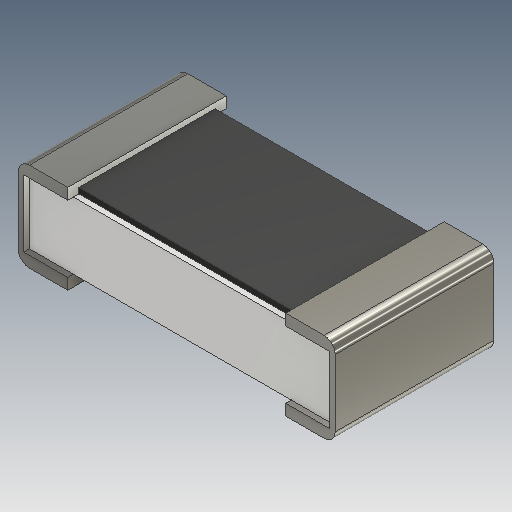
# Autodesk Inventor part: RC0603
Saved by Autodesk Inventor 2018 (Build 220112000, 112)
## iProperties
Created: 2015-10-12
Part Number: RC0603
Material: ABS Plastic
Document SubType Name: Modeling
Designer: Sawaiz
Density: 1.06 g/cm^3
Appearance: Smooth - White
Author: Sawaiz
Autodesk Inventor part; units mm, degrees
ref_plane "YZ Plane" through (0, 0, 0) normal (1, 0, 0) x (0, 1, 0)
ref_plane "XZ Plane" through (0, 0, 0) normal (0, 1, 0) x (-1, 0, 0)
ref_plane "XY Plane" through (0, 0, 0) normal (0, 0, 1) x (1, 0, 0)
sketch "Sketch1" plane through (0, 0, 0) normal (0, 0, 1) x (1, 0, 0)
  line L0 (0.4, -0.8) -> (-0.4, -0.8)
  line L1 (-0.4, -0.8) -> (-0.4, 0.8)
  line L2 (-0.4, 0.8) -> (0.4, 0.8)
  line L3 (0.4, 0.8) -> (0.4, -0.8)
  line L4 (0.4, -0.8) -> (-0.4, 0.8) construction
  line L5 (-0.4, -0.8) -> (0.4, 0.8) construction
  point P0 (0, 0)
  dimension "d0" = 0.8
  dimension "d1" = 1.6
  constraints: 12 end point, 2 midpoint, 2 parallel, 1 horizontal, 1 perpendicular
  measures "d0" distance of L1.end L2.end
  measures "d1" distance of L0.end L1.end
extrude "Extrusion1" add sketch "Sketch1" along normal blind 0.45
sketch "Sketch2" plane through (0, 0, 0) normal (0, 0, -1) x (-1, 0, 0)
  line L0 (-0.4, -0.8) -> (0.4, -0.8) projected
  line L1 (0.4, -0.8) -> (0.4, 0.8) projected
  line L2 (0.4, 0.8) -> (-0.4, 0.8) projected
  line L3 (-0.4, 0.8) -> (-0.4, -0.8) projected
  line L4 (-0.4, -0.55) -> (0.4, -0.55)
  line L5 (0.4, 0.8) -> (0.4, -0.8) projected
  line L6 (0.4, 0.55) -> (-0.4, 0.55)
  point P0 (0, 0)
  dimension "d4" = 0.25
  dimension "d5" = 0.25
  constraints: 4 end point, 4 point on line, 1 horizontal, 1 parallel
  measures "d4" distance between parallel lines of L2 L6
  measures "d5" distance between parallel lines of L0 L4
extrude "Extrusion2" cut sketch "Sketch2" against normal blind 0.0563 contours L3 L6 L1 L4
sketch "Sketch3" plane through (0, 0, 0.45) normal (0, 0, 1) x (1, 0, 0)
  line L0 (-0.4, -0.8) -> (0.4, -0.8) projected
  line L1 (0.4, -0.8) -> (0.4, 0.8) projected
  line L2 (0.4, 0.8) -> (-0.4, 0.8) projected
  line L3 (-0.4, 0.8) -> (-0.4, -0.8) projected
  line L4 (-0.4, 0.55) -> (-0.4, -0.55) projected
  line L5 (-0.4, -0.8) -> (-0.4, 0.8) projected
  line L6 (0.4, 0.8) -> (-0.4, 0.8) projected
  line L7 (0.4, 0.55) -> (-0.4, 0.55)
  line L8 (-0.4, 0.55) -> (-0.4, -0.55)
  line L9 (-0.4, -0.55) -> (0.4, -0.55)
  line L10 (0.4, -0.55) -> (0.4, 0.55)
  line L11 (0.4, 0.55) -> (-0.4, -0.55) construction
  line L12 (-0.4, 0.55) -> (0.4, -0.55) construction
  point P0 (0, 0)
  dimension "d22" = 0.25
  constraints: 12 end point, 2 midpoint, 2 parallel, 1 horizontal, 1 perpendicular, 1 point on line
  measures "d22" distance between parallel lines of L0 L9
extrude "Extrusion7" cut sketch "Sketch3" against normal blind 0.0563 contours L3 L7 L1 L9
sketch "Sketch4" plane through (0.4, -0.8, 0.45) normal (1, 0, 0) x (0, 0, -1)
  line L0 (0, 0) -> (0, 0.25) projected
  line L1 (0.45, 0) -> (0, 0) projected
  line L2 (0.45, 0.25) -> (0.45, 0) projected
  line L3 (0.45, 1.6) -> (0, 1.6) projected
  line L4 (0.45, 0.25) -> (0.3938, 0.25) projected
  line L5 (0.3938, 0.25) -> (0.3938, 1.35) projected
  line L6 (0.3938, 1.35) -> (0.45, 1.35) projected
  line L7 (0.45, 1.6) -> (0.45, 1.35) projected
  line L8 (0.0562, 0.25) -> (0, 0.25) projected
  line L9 (0, 1.35) -> (0.0562, 1.35) projected
  line L10 (0.0562, 1.35) -> (0.0562, 0.25) projected
  line L11 (0.3938, 0.0281) -> (0.0562, 0.0281)
  line L12 (0.0562, 0.0281) -> (0.0562, 1.5719)
  line L13 (0.0562, 1.5719) -> (0.3937, 1.5719)
  line L14 (0.3937, 1.5719) -> (0.3938, 0.0281)
  line L15 (0.3938, 0.0281) -> (0.0562, 1.5719) construction
  line L16 (0.0562, 0.0281) -> (0.3937, 1.5719) construction
  line L17 (0, 1.35) -> (0, 1.6) projected
  point P0 (0.225, 0.8)
  dimension "d25" = 0.0281
  dimension "d26" = 0.0281
  constraints: 12 end point, 2 collinear, 2 midpoint, 2 parallel, 1 horizontal, 1 perpendicular
  measures "d25" distance between parallel lines of L3 L13
  measures "d26" distance between parallel lines of L1 L11
extrude "Extrusion8" cut sketch "Sketch4" against normal blind 0.0281 contours L10 L12 L13 L14 L5 L11
mirror "Mirror1" about plane through (0, 0, 0) normal (1, 0, 0) of "Extrusion8"
sketch "Sketch7" plane through (0, 0, 0.3938) normal (0, 0, 1) x (1, 0, 0)
  line L0 (-0.3719, 0.55) -> (-0.3719, -0.55) projected
  line L1 (0.3719, -0.55) -> (-0.3719, -0.55) projected
  line L2 (0.3719, -0.55) -> (0.3719, 0.55) projected
  line L3 (-0.3719, 0.55) -> (0.3719, 0.55) projected
  point P0 (0, 0)
extrude "Extrusion9" add sketch "Sketch7" along normal blind 0.0281
sketch "Sketch8" plane through (0.3719, -0.8, 0.45) normal (1, 0, 0) x (0, 0, -1)
  line L0 (0.3938, 0.0281) -> (0.0562, 0.0281) projected
  line L1 (0.3938, 0.25) -> (0.3938, 0.0281) projected
  line L2 (0.3937, 1.35) -> (0.3938, 0.25) projected
  line L3 (0.3937, 1.5719) -> (0.3937, 1.35) projected
  line L4 (0.0562, 1.5719) -> (0.3937, 1.5719) projected
  line L5 (0.0562, 1.35) -> (0.0562, 1.5719) projected
  line L6 (0.0281, 1.35) -> (0.0562, 1.35) projected
  line L7 (0.0281, 0.25) -> (0.0281, 1.35) projected
  line L8 (0.0562, 0.25) -> (0.0281, 0.25) projected
  line L9 (0.0562, 0.0281) -> (0.0562, 0.25) projected
  line L10 (0.0562, 0.25) -> (0.0562, 1.35)
  point P0 (0.45, 0.8)
  constraints: 2 end point, 1 vertical
extrude "Extrusion10" cut sketch "Sketch8" against normal blind 0.0281 contours L8 L7 L6 L10
mirror "Mirror2" about plane through (0, 0, 0) normal (1, 0, 0) of "Extrusion10"
fillet "Fillet1" radius 0.0563 4 edges at (0, -0.8, 0.45) (0, 0.8, 0.45) (0, 0.8, 0) (0, -0.8, 0)
equation "\"d0\" = width"
equation "\"d1\" = length"
equation "\"d2\" = height"
equation "\"d4\" = i2"
equation "\"d5\" = i2"
equation "\"d6\" = 0.125 * height"
equation "\"d22\" = i1"
equation "\"d23\" = 0.125 * height"
equation "\"d25\" = 0.0625 * height"
equation "\"d26\" = 0.0625 * height"
equation "\"d27\" = 0.0625 * height"
equation "\"d29\" = 0.0625 * height"
equation "\"d31\" = 0.0625 * height"
equation "\"d21\" = 0.125 * height"
equation "\"length\" = 1.6"
equation "\"width\" = 0.8"
equation "\"height\" = 0.45"
equation "\"i1\" = 0.25"
equation "\"i2\" = 0.25"
body "Solid1"
